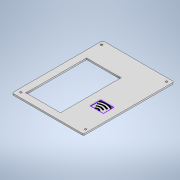
# Autodesk Inventor part: frontpanel
Saved by Autodesk Inventor 2022 (Build 260153000, 153)
## iProperties
Created: 2022-02-23
Part Number: frontpanel
Material: Generisch
Document SubType Name: Modeling
Designer: ga76xid
Density: 1 g/cm^3
Appearance: Vorgabe
Author: ga76xid
Autodesk Inventor part; units mm, degrees
ref_plane "YZ Plane" through (0, 0, 0) normal (1, 0, 0) x (0, 1, 0)
ref_plane "XZ Plane" through (0, 0, 0) normal (0, 1, 0) x (-1, 0, 0)
sketch "Skizze1" plane through (0, 0, 0) normal (0, 1, 0) x (-1, 0, 0)
  line L0 (0, 0) -> (-90, 0)
  line L1 (-90, 0) -> (-90, -158)
  line L2 (-90, -158) -> (0, -158)
  line L3 (0, -158) -> (0, 0)
  line L4 (18, 18) -> (-168, 18)
  line L5 (-168, 18) -> (-168, -218)
  line L6 (-168, -218) -> (18, -218)
  line L7 (18, -218) -> (18, 18)
  circle A0 centre (8, 5.5) radius 2.5
  circle A1 centre (10, -207) radius 2.5
  circle A2 centre (-158, -208.5) radius 2.5
  circle A3 centre (-160, 4.5) radius 2.5
  dimension "d0" = 90
  dimension "d1" = 158
  dimension "d2" = 78
  dimension "d3" = 18
  dimension "d4" = 18
  dimension "d5" = 60
  dimension "r" = 5
  dimension "d7" = 5
  dimension "d8" = 5
  dimension "d9" = 5
  dimension "d10" = 8
  dimension "d11" = 5.5
  dimension "d12" = 4.5
  dimension "d13" = 70
  dimension "d14" = 68
  dimension "d15" = 50.5
  dimension "d16" = 49
  dimension "d17" = 10
  constraints: 16 end point, 4 centre point, 4 parallel, 2 horizontal, 2 perpendicular
  measures "d0" distance of L2.end L1.end
  measures "d1" distance of L1.end L0.end
  measures "d2" distance between parallel lines of L5 L1
  measures "d3" distance between parallel lines of L4 L0
  measures "d4" distance between parallel lines of L7 L3
  measures "d5" distance between parallel lines of L2 L6
  measures "r" diameter of A0
  measures "d7" diameter of A1
  measures "d8" diameter of A2
  measures "d9" diameter of A3
  measures "d10" distance from line of L3 A0.centre
  measures "d11" distance from line of L0 A0.centre
  measures "d12" distance from line of L0 A3.centre
  measures "d13" distance from line of L1 A3.centre
  measures "d14" distance from line of A2.centre L1
  measures "d15" distance from line of L2 A2.centre
  measures "d16" distance from line of L2 A1.centre
  measures "d17" distance from line of L3 A1.centre
extrude "Extrusion1" add sketch "Skizze1" along normal blind 4
fillet "Rundung1" radius 3 4 edges at (-18, 2, -218) (-18, 2, 18) (168, 2, 18) (168, 2, -218)
ref_plane "Arbeitsebene1" through (0, 8, 0) normal (0, 1, 0) x (1, 0, 0)
sketch "Skizze3" plane through (0, 4, 0) normal (0, 1, 0) x (1, 0, 0)
  line L0 (112.9385, 54.4149) -> (112.9385, 81.7299)
  line L1 (112.9385, 81.7299) -> (146.9954, 81.7299) construction
  line L2 (146.9954, 81.7299) -> (146.9954, 54.4149) construction
  line L3 (146.9954, 54.4149) -> (112.9385, 54.4149) construction
  line L4 (112.9385, 54.4149) -> (146.9954, 54.4149)
  line L5 (146.9954, 54.4149) -> (146.9954, 81.7299)
  line L6 (146.9954, 81.7299) -> (112.9385, 81.7299)
  line L7 (112.9385, 81.7299) -> (112.9385, 54.4149)
  point P0 (0, 0)
  constraints: 8 end point, 2 parallel, 1 horizontal, 1 perpendicular, 1 vertical, 2 other
extrude "Extrusion3" cut sketch "Skizze3" against normal blind 2
equation "\"d7\" = r"
equation "\"d8\" = r"
equation "\"d9\" = r"
equation "\"d50\" = a"
equation "\"d51\" = a"
equation "\"d52\" = a"
equation "\"a\" = 2.6"
